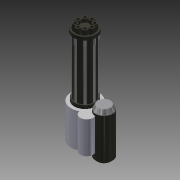
# Autodesk Inventor part: gatling
Saved by Autodesk Inventor 2014 (Build 180170000, 170)
## iProperties
Created: 2017-01-04
Part Number: gatling
Material: Generic
Document SubType Name: Modeling
Designer: potato
Density: 1 g/cm^3
Appearance: Default
Author: potato
Autodesk Inventor part; units mm, degrees
ref_plane "YZ Plane" through (0, 0, 0) normal (1, 0, 0) x (0, 1, 0)
sketch "Sketch1" plane through (0, 0, 0) normal (0, 1, 0) x (-1, 0, 0)
  circle A0 centre (0, 0) radius 133.35
  circle A1 centre (0, 0) radius 114.3
  dimension "d40" = 266.7
  dimension "d41" = 228.6
  constraints: 2 centre point, 2 coincident
  measures "d40" diameter of A0
  measures "d41" diameter of A1
extrude "Extrusion1" add sketch "Sketch1" along normal blind 38.1
sketch "Sketch3" plane through (0, 0, 0) normal (0, -1, 0) x (1, 0, 0)
  circle A0 centre (0, 0) radius 114.3 projected
  circle A1 centre (0, 0) radius 133.35 projected
  circle A2 centre (0, 0) radius 114.3
  constraints: 1 centre point, 1 coincident, 1 concentric
extrude "Extrusion2" add sketch "Sketch3" against normal blind 12.7 contours A0
sketch "Sketch4" plane through (0, 12.7, 0) normal (0, 1, 0) x (1, 0, 0)
  circle A0 centre (0, 0) radius 114.3 projected
  circle A1 centre (0, 0) radius 50.8
  dimension "d9" = 101.6
  constraints: 1 centre point, 1 coincident
  measures "d9" diameter of A1
extrude "Extrusion4" add sketch "Sketch4" along normal blind 44.45 contours A1
sketch "Sketch5" plane through (0, 12.7, 0) normal (0, 1, 0) x (1, 0, 0)
  circle A0 centre (0, 0) radius 114.3 projected
  circle A1 centre (0, 0) radius 82.55
  circle A2 centre (-82.55, 0) radius 28.575
  circle A3 centre (82.55, 0) radius 28.575
  circle A4 centre (0, 82.55) radius 28.575
  circle A5 centre (0, -82.55) radius 28.575
  circle A6 centre (-58.3717, -58.3717) radius 28.575
  circle A7 centre (58.3717, -58.3717) radius 28.575
  line L0 (-82.55, 0) -> (82.55, 0)
  circle A8 centre (-58.3717, 58.3717) radius 28.575
  circle A9 centre (58.3717, 58.3717) radius 28.575
  circle A10 centre (-82.55, 0) radius 15.875
  circle A11 centre (-58.3717, 58.3717) radius 15.875
  circle A12 centre (0, 82.55) radius 15.875
  circle A13 centre (58.3717, 58.3717) radius 15.875
  circle A14 centre (82.55, 0) radius 15.875
  circle A15 centre (58.3717, -58.3717) radius 15.875
  circle A16 centre (0, -82.55) radius 15.875
  circle A17 centre (-58.3717, -58.3717) radius 15.875
  dimension "d12" = 165.1
  dimension "d13" = 57.15
  dimension "d14" = 57.15
  dimension "d15" = 57.15
  dimension "d16" = 57.15
  dimension "d17" = 57.15
  dimension "d18" = 57.15
  dimension "d19" = 31.75
  dimension "d20" = 31.75
  dimension "d21" = 31.75
  dimension "d22" = 31.75
  dimension "d23" = 31.75
  dimension "d24" = 31.75
  dimension "d25" = 31.75
  dimension "d26" = 31.75
  constraints: 17 centre point, 9 coincident, 6 point on circle, 2 end point, 2 symmetric about line, 1 horizontal, 2 other
  measures "d12" diameter of A1
  measures "d13" diameter of A2
  measures "d14" diameter of A3
  measures "d15" diameter of A4
  measures "d16" diameter of A5
  measures "d17" diameter of A6
  measures "d18" diameter of A7
  measures "d19" diameter of A10
  measures "d20" diameter of A11
  measures "d21" diameter of A12
  measures "d22" diameter of A13
  measures "d23" diameter of A14
  measures "d24" diameter of A15
  measures "d25" diameter of A16
  measures "d26" diameter of A17
extrude "Extrusion5" add sketch "Sketch5" along normal blind 76.2 and the other way blind 700 contours A14 L0 A3 A1 | A1 A3 A14 | A1 A3 L0 A14 | A9 A1 A13 | A1 A13 A9 | A7 A1 A15 | A1 A15 A7 | L0 A10 A1 A2 | A2 A1 A10 L0 | A1 A10 A2 | A4 A1 A12 | A1 A12 A4 | A5 A1 A16 | A1 A16 A5 | A8 A1 A11 | A1 A11 A8 | A6 A1 A17 | A1 A17 A6
sketch "Sketch7" plane through (0, 0, 0) normal (0, -1, 0) x (1, 0, 0)
  circle A0 centre (58.3717, -58.3717) radius 28.575
  circle A1 centre (58.3717, 58.3717) radius 28.575
  circle A2 centre (0, 82.55) radius 28.575
  circle A3 centre (82.55, 0) radius 28.575
  circle A4 centre (-82.55, 0) radius 28.575
  circle A5 centre (0, -82.55) radius 28.575
  circle A6 centre (-58.3717, 58.3717) radius 28.575
  circle A7 centre (-58.3717, -58.3717) radius 28.575
  circle A8 centre (0, 0) radius 139.7
  circle A9 centre (0, 0) radius 111.125
  circle A10 centre (58.3717, -58.3717) radius 28.575 projected
  circle A11 centre (58.3717, 58.3717) radius 28.575 projected
  circle A12 centre (0, 82.55) radius 28.575 projected
  circle A13 centre (82.55, 0) radius 28.575 projected
  circle A14 centre (-82.55, 0) radius 28.575 projected
  circle A15 centre (0, -82.55) radius 28.575 projected
  circle A16 centre (-58.3717, 58.3717) radius 28.575 projected
  circle A17 centre (-58.3717, -58.3717) radius 28.575 projected
  circle A18 centre (0, 0) radius 133.35 projected
  dimension "d37" = 222.25
  constraints: 10 centre point, 1 coincident
  measures "d37" diameter of A9
sketch "Sketch8" plane through (82.55, -687.3, 0) normal (0, -1, 0) x (1, 0, 0)
  circle A0 centre (-82.55, 0) radius 127
  dimension "d32" = 254
  constraints: 1 centre point, 1 coincident
  measures "d32" diameter of A0
extrude "Extrusion6" add sketch "Sketch8" along normal blind 25.4 and the other way blind 12.7
sketch "Sketch9" plane through (0, 0, 0) normal (0, -1, 0) x (1, 0, 0)
  line L0 (0, 0) -> (131.7027, 0) construction
  line L1 (0, 0) -> (139.7, 0) construction
  line L2 (0, 0) -> (139.7, 0) construction
  line L3 (0, 0) -> (139.7, 0) construction
  line L4 (0, 0) -> (139.7, 0) construction
  line L5 (0, 0) -> (139.7, 0) construction
  line L6 (0, 0) -> (139.7, 0) construction
  line L7 (0, 0) -> (139.7, 0) construction
  line L8 (0, 0) -> (139.7, 0) construction
  line L9 (0, 0) -> (139.7, 0) construction
  line L10 (-103.3862, 93.7038) -> (-103.5109, 93.8168)
  line L11 (-110.1743, -14.5047) -> (-126.847, -6.2316)
  line L12 (-126.8485, 6.2019) -> (-110.1743, 14.5047)
  arc A0 (-85.31, 94.0808) -> (-94.1008, 85.288) centre (0, 0) ccw
  line L13 (-67.6486, -88.1614) -> (-85.288, -94.1008)
  line L14 (-94.0808, -85.31) -> (-88.1614, -67.6486)
  line L15 (-6.2019, -126.8485) -> (-14.5047, -110.1743)
  line L16 (14.5047, -110.1743) -> (6.2316, -126.847)
  line L17 (85.31, -94.0808) -> (67.6486, -88.1614)
  line L18 (88.1614, -67.6486) -> (94.1008, -85.288)
  line L19 (126.8485, -6.2019) -> (110.1743, -14.5047)
  line L20 (110.1743, 14.5047) -> (126.847, 6.2316)
  line L21 (94.0808, 85.31) -> (88.1614, 67.6486)
  line L22 (67.6486, 88.1614) -> (85.288, 94.1008)
  line L23 (-14.5047, 110.1743) -> (-6.2316, 126.847)
  line L24 (6.2019, 126.8485) -> (14.5047, 110.1743)
  line L25 (-88.1614, 67.6486) -> (-94.1008, 85.288)
  line L26 (-85.31, 94.0808) -> (-67.6486, 88.1614)
  arc A1 (-126.8485, 6.2019) -> (-126.847, -6.2316) centre (0, 0) ccw
  arc A2 (-94.0808, -85.31) -> (-85.288, -94.1008) centre (0, 0) ccw
  arc A3 (-6.2019, -126.8485) -> (6.2316, -126.847) centre (0, 0) ccw
  arc A4 (85.31, -94.0808) -> (94.1008, -85.288) centre (0, 0) ccw
  arc A5 (126.8485, -6.2019) -> (126.847, 6.2316) centre (0, 0) ccw
  arc A6 (94.0808, 85.31) -> (85.288, 94.1008) centre (0, 0) ccw
  arc A7 (6.2019, 126.8485) -> (-6.2316, 126.847) centre (0, 0) ccw
  arc A8 (-67.6486, 88.1614) -> (-88.1614, 67.6486) centre (0, 0) ccw
  circle A9 centre (0, 0) radius 111.125
  arc A10 (-126.8485, 6.2019) -> (-126.847, -6.2316) centre (0, 0) ccw
  arc A11 (-110.1743, 14.5047) -> (-110.1743, -14.5047) centre (0, 0) ccw
  arc A12 (-88.1614, -67.6486) -> (-67.6486, -88.1614) centre (-0.0002, -0.0002) ccw
  arc A13 (-94.0808, -85.31) -> (-85.288, -94.1008) centre (0, 0) ccw
  arc A14 (-14.5047, -110.1743) -> (14.5047, -110.1743) centre (0, -0.0004) ccw
  arc A15 (-6.2019, -126.8485) -> (6.2316, -126.847) centre (0, 0) ccw
  arc A16 (67.6486, -88.1614) -> (88.1614, -67.6486) centre (0.0004, -0.0004) ccw
  arc A17 (85.31, -94.0808) -> (94.1008, -85.288) centre (0, 0) ccw
  arc A18 (110.1743, -14.5047) -> (110.1743, 14.5047) centre (0.0002, 0) ccw
  arc A19 (126.8485, -6.2019) -> (126.847, 6.2316) centre (0, 0) ccw
  arc A20 (88.1614, 67.6486) -> (67.6486, 88.1614) centre (0.0002, 0.0002) ccw
  arc A21 (94.0808, 85.31) -> (85.288, 94.1008) centre (0, 0) ccw
  arc A22 (14.5047, 110.1743) -> (-14.5047, 110.1743) centre (0, 0.0001) ccw
  arc A23 (6.2019, 126.8485) -> (-6.2316, 126.847) centre (0, 0) ccw
  arc A24 (126.8485, -6.2019) -> (126.847, 6.2316) centre (0, 0) ccw
  arc A25 (110.1743, -14.5047) -> (110.1743, 14.5047) centre (0.0002, 0) ccw
  constraints: 54 end point, 53 point on circle, 26 centre point, 10 horizontal, 1 coincident
extrude "Extrusion8" add sketch "Sketch9" along normal blind 76.2 contours L11 A1 L12 A9 | A9 L13 A2 L14 | L25 A0 L26 A8 | A9 L16 A3 L15 | L23 A7 L24 A9 | A9 L18 A4 L17 | L22 A6 L21 A9 | A9 L20 A5 L19
extrude "Extrusion9" add sketch "Sketch7" along normal blind 675.64 contours A9
sketch "Sketch10" plane through (0, -76.2, 0) normal (0, -1, 0) x (1, 0, 0)
  line L0 (-126.847, -6.2316) -> (-110.1743, -14.5047) projected
  arc A0 (-110.1743, 14.5047) -> (-110.1743, -14.5047) centre (0, 0) ccw projected
  line L1 (-110.1743, 14.5047) -> (-126.8485, 6.2019) projected
  line L2 (-118.5114, 10.3533) -> (-110.1743, 14.5047)
  line L3 (-114.3429, 12.429) -> (-114.342, -12.4367)
  constraints: 4 end point, 2 midpoint, 1 collinear, 1 point on line
extrude "Extrusion10" add sketch "Sketch10" along normal blind 599.44
sketch "Sketch11" plane through (0, -76.2, 0) normal (0, -1, 0) x (1, 0, 0)
  line L0 (-67.6486, 88.1614) -> (-85.31, 94.0808) projected
  line L1 (-94.1008, 85.288) -> (-88.1614, 67.6486) projected
  arc A0 (-67.6486, 88.1614) -> (-88.1614, 67.6486) centre (0, 0) ccw projected
  line L2 (-88.1614, 67.6486) -> (-89.6447, 72.0538)
  line L3 (-67.6486, 88.1614) -> (-72.0559, 89.6385)
  line L4 (-72.0559, 89.6385) -> (-89.6447, 72.0538)
  dimension "d59" = 4.6482
  dimension "d60" = 4.6482
  constraints: 6 end point, 2 point on line
  measures "d59" distance of L1.end L2.end
  measures "d60" distance of L0.start L3.end
extrude "Extrusion11" add sketch "Sketch11" along normal blind 599.44
sketch "Sketch12" plane through (0, -76.2, 0) normal (0, -1, 0) x (1, 0, 0)
  arc A0 (14.5047, 110.1743) -> (-14.5047, 110.1743) centre (0, 0.0001) ccw projected
  line L0 (14.5047, 110.1743) -> (6.2019, 126.8485) projected
  line L1 (-6.2316, 126.847) -> (-14.5047, 110.1743) projected
  line L2 (-14.5047, 110.1743) -> (-12.4386, 114.3381)
  line L3 (14.5047, 110.1743) -> (12.4314, 114.3381)
  line L4 (-12.4386, 114.3381) -> (12.4314, 114.3381)
  dimension "d63" = 4.6482
  constraints: 6 end point, 2 point on line, 1 horizontal
  measures "d63" distance of L1.end L2.end
sketch "Sketch13" plane through (0, -76.2, 0) normal (0, -1, 0) x (1, 0, 0)
  arc A0 (88.1614, 67.6486) -> (67.6486, 88.1614) centre (0.0002, 0.0002) ccw projected
  line L0 (88.1614, 67.6486) -> (94.0808, 85.31) projected
  line L1 (85.288, 94.1008) -> (67.6486, 88.1614) projected
  line L2 (67.6486, 88.1614) -> (72.0538, 89.6447)
  line L3 (72.0538, 89.6447) -> (89.6385, 72.0559)
  line L4 (88.1614, 67.6486) -> (89.6385, 72.0559)
  line L5 (89.6385, 72.0559) -> (72.0538, 89.6447)
  dimension "d64" = 4.6482
  dimension "d65" = 4.6482
  constraints: 8 end point, 3 point on line, 1 collinear
  measures "d64" distance of L1.end L2.end
  measures "d65" distance of L0.start L4.end
sketch "Sketch14" plane through (0, -76.2, 0) normal (0, -1, 0) x (1, 0, 0)
  line L0 (110.1743, -14.5047) -> (126.8485, -6.2019) projected
  line L1 (126.847, 6.2316) -> (110.1743, 14.5047) projected
  arc A0 (110.1743, -14.5047) -> (110.1743, 14.5047) centre (0.0002, 0) ccw projected
  line L2 (110.1743, 14.5047) -> (114.3381, 12.4386)
  line L3 (114.3381, 12.4386) -> (114.3381, -12.4314)
  line L4 (110.1743, -14.5047) -> (114.3381, -12.4314)
  dimension "d66" = 4.6482
  constraints: 6 end point, 2 point on line, 1 collinear, 1 vertical
  measures "d66" distance of L1.end L2.end
sketch "Sketch15" plane through (0, -76.2, 0) normal (0, -1, 0) x (1, 0, 0)
  line L0 (-85.288, -94.1008) -> (-67.6486, -88.1614) projected
  arc A0 (-88.1614, -67.6486) -> (-67.6486, -88.1614) centre (-0.0002, -0.0002) ccw projected
  line L1 (-88.1614, -67.6486) -> (-94.0808, -85.31) projected
  line L2 (-88.1614, -67.6486) -> (-89.6385, -72.0559)
  line L3 (-67.6486, -88.1614) -> (-72.0538, -89.6447)
  line L4 (-72.0538, -89.6447) -> (-89.6385, -72.0559)
  dimension "d67" = 4.6482
  dimension "d68" = 4.6482
  constraints: 6 end point, 2 point on line
  measures "d67" distance of L1.start L2.end
  measures "d68" distance of L0.end L3.end
sketch "Sketch16" plane through (0, -76.2, 0) normal (0, -1, 0) x (1, 0, 0)
  line L0 (6.2316, -126.847) -> (14.5047, -110.1743) projected
  arc A0 (-14.5047, -110.1743) -> (14.5047, -110.1743) centre (0, -0.0004) ccw projected
  line L1 (-14.5047, -110.1743) -> (-6.2019, -126.8485) projected
  line L2 (14.5047, -110.1743) -> (12.4386, -114.3381)
  line L3 (12.4386, -114.3381) -> (-12.4314, -114.3381)
  line L4 (-14.5047, -110.1743) -> (-12.4314, -114.3381)
  dimension "d69" = 4.6482
  constraints: 6 end point, 2 point on line, 1 collinear, 1 horizontal
  measures "d69" distance of L0.end L2.end
sketch "Sketch17" plane through (0, -76.2, 0) normal (0, -1, 0) x (1, 0, 0)
  line L0 (94.1008, -85.288) -> (88.1614, -67.6486) projected
  arc A0 (67.6486, -88.1614) -> (88.1614, -67.6486) centre (0.0004, -0.0004) ccw projected
  line L1 (67.6486, -88.1614) -> (85.31, -94.0808) projected
  line L2 (88.1614, -67.6486) -> (89.6447, -72.0538)
  line L3 (67.6486, -88.1614) -> (72.0559, -89.6385)
  line L4 (72.0559, -89.6385) -> (89.6447, -72.0538)
  dimension "d70" = 4.6482
  dimension "d71" = 4.6482
  constraints: 6 end point, 2 point on line
  measures "d70" distance of L0.end L2.end
  measures "d71" distance of L1.start L3.end
extrude "Extrusion12" add sketch "Sketch16" along normal blind 599.44
extrude "Extrusion13" add sketch "Sketch15" along normal blind 599.44
extrude "Extrusion14" add sketch "Sketch17" along normal blind 599.44
extrude "Extrusion15" add sketch "Sketch14" along normal blind 599.44
extrude "Extrusion16" add sketch "Sketch12" along normal blind 599.44
extrude "Extrusion17" add sketch "Sketch13" along normal blind 599.44
sketch "Sketch25" plane through (72.0559, -674.6, -89.6385) normal (0.7070249, 0, -0.7071887) x (-0.7071887, 0, -0.7070249)
  line L0 (0, 0) -> (-24.8715, 0) projected
  line L1 (-24.8715, 0) -> (-18.2555, 37.5212)
  line L2 (-24.8715, 0) -> (13.2285, 0) construction
  line L3 (0, 0) -> (-6.616, 37.5212)
  line L4 (0, 0) -> (38.1, 0) construction
  line L5 (-6.616, 37.5212) -> (-18.2555, 37.5212)
  point P0 (-12.4196, 674.6)
  dimension "d115" = 38.1
  dimension "d116" = 80
  dimension "d117" = 38.1
  dimension "d118" = 100
  constraints: 10 end point, 2 equal length, 2 horizontal
  measures "d115" distance of L0.end L1.end
  measures "d116" angle of L2 L1
  measures "d117" distance of L0.start L3.end
  measures "d118" angle of L4 L3
extrude "Extrusion22" add sketch "Sketch25" along normal blind 12.7
sketch "Sketch26" plane through (72.0559, -674.6, -89.6385) normal (0.7070249, 0, -0.7071887) x (-0.7071887, 0, -0.7070249)
  line L0 (-24.8715, 0) -> (0, 0)
  line L1 (0, 0) -> (0, 50.8)
  line L2 (0, 50.8) -> (-24.8715, 50.8)
  line L3 (-24.8715, 50.8) -> (-24.8715, 0)
  dimension "d121" = 50.8
  constraints: 8 end point, 2 parallel, 1 horizontal, 1 perpendicular
  measures "d121" distance of L1.end L0.end
loft "Loft3" add profiles "Sketch26" section 2 edges at (89.8295, -674.6, -89.8275) (83.3745, -655.8394, -96.281) (89.8295, -637.0788, -89.8275) (96.2845, -655.8394, -83.3739)
sketch "Sketch28" plane through (0, -712.7, 0) normal (0, -1, 0) x (1, 0, 0)
  circle A0 centre (0, 0) radius 127 projected
  circle A1 centre (0, 0) radius 165.1
  dimension "d126" = 330.2
  constraints: 1 centre point, 1 coincident
  measures "d126" diameter of A1
extrude "Extrusion23" add sketch "Sketch28" along normal blind 406.4 contours A0 | A1
sketch "Sketch33" plane through (0, -1119.1, 0) normal (0, -1, 0) x (1, 0, 0)
  circle A0 centre (228.6, 0) radius 101.6
  constraints: 1 centre point
extrude "Extrusion25" add sketch "Sketch33" along normal blind 50.8 and the other way blind 431.8
ref_plane "Work Plane6" through (228.6, -636.5, 0) normal (0, 1, 0) x (1, 0, 0)
sketch "Sketch35" plane through (228.6, -636.5, 0) normal (0, 1, 0) x (1, 0, 0)
  circle A0 centre (0, 0) radius 76.2
  point P0 (-228.6, 0)
  dimension "d146" = 152.4
  constraints: 1 centre point
  measures "d146" diameter of A0
loft "Loft5" add profiles "Sketch35" section 2 edges at (228.6, -687.3, -101.6) (228.6, -687.3, 101.6)
ref_plane "Work Plane7" through (228.6, -1195.3, 0) normal (0, -1, 0) x (1, 0, 0)
sketch "Sketch36" plane through (228.6, -1195.3, 0) normal (0, -1, 0) x (1, 0, 0)
  circle A0 centre (0, 0) radius 76.2
  point P0 (-228.6, 0)
  dimension "d152" = 152.4
  constraints: 1 centre point
  measures "d152" diameter of A0
loft "Loft6" add profiles "Sketch36" section 1 edges at (127, -1169.9, 0)
sketch "Sketch37" plane through (0, -1119.1, 0) normal (0, -1, 0) x (1, 0, 0)
  arc A0 (151.3417, 65.9826) -> (151.3417, -65.9826) centre (0, 0) ccw projected
  circle A1 centre (0, 0) radius 127
  dimension "d157" = 254
  constraints: 1 centre point, 1 coincident
  measures "d157" diameter of A1
extrude "Extrusion26" add sketch "Sketch37" along normal blind 25.4
sketch "Sketch38" plane through (0, -1119.1, 0) normal (0, -1, 0) x (1, 0, 0)
  circle A0 centre (0, 0) radius 127 projected
  circle A1 centre (153.8111, 132.787) radius 76.2
  circle A2 centre (228.6, 0) radius 101.6 projected
  circle A3 centre (228.6, 0) radius 76.2 projected
  dimension "d160" = 152.4
  constraints: 2 tangent, 1 centre point
  measures "d160" diameter of A1
extrude "Extrusion27" add sketch "Sketch38" against normal blind 406.4 contours A1 A2 | A2 A1 picked at (157.9557, 125.2358) picked at (182.9676, 81.02)
sketch "Sketch39" plane through (0, -1119.1, 0) normal (0, -1, 0) x (1, 0, 0)
  arc A0 (223.2739, 101.4603) -> (127, 0) centre (228.6, 0) ccw projected
  arc A1 (223.2739, 101.4603) -> (78.625, 145.1762) centre (153.8111, 132.787) ccw projected
  arc A2 (144.5949, 57.1464) -> (78.625, 145.1762) centre (153.8111, 132.787) ccw
  circle A3 centre (0, 0) radius 165.1
  arc A4 (155.0958, 56.5978) -> (78.625, 145.1762) centre (0, 0) ccw
  constraints: 9 point on circle, 3 centre point, 1 coincident, 1 concentric
extrude "Extrusion28" cut sketch "Sketch39" against normal blind 25.4 contours A2 A3 A0 | A0 A3 A1 picked at (181.9563, 80.4364)
sketch "Sketch40" plane through (0, -1119.1, 0) normal (0, 1, 0) x (1, 0, 0)
  arc A0 (151.3417, -65.9826) -> (223.2739, -101.4603) centre (228.6, 0) ccw projected
  arc A1 (223.2739, -101.4603) -> (155.0958, -56.5978) centre (153.8111, -132.787) ccw projected
  arc A2 (151.3417, -65.9826) -> (155.0958, -56.5978) centre (0, 0) ccw projected
extrude "Extrusion29" add sketch "Sketch40" along normal blind 25.4
body "Solid1"
